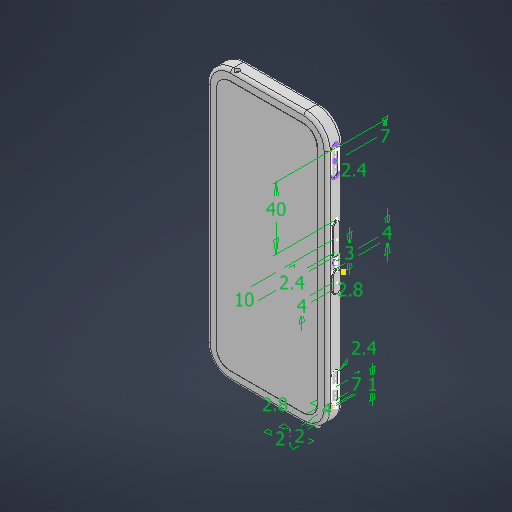
# Autodesk Inventor part: proiect_modelare3D
Saved by Autodesk Inventor 2026.2 (Build 302298000, 298)
## iProperties
Created: 2026-01-05
Part Number: proiect_modelare3D
Material: Generic
Document SubType Name: Modeling
Designer: laura
Density: 1 g/cm^3
Appearance: Default
Author: laura
Autodesk Inventor part; units mm, degrees
ref_plane "YZ Plane" through (0, 0, 0) normal (1, 0, 0) x (0, 1, 0)
ref_plane "XZ Plane" through (0, 0, 0) normal (0, 1, 0) x (-1, 0, 0)
ref_plane "XY Plane" through (0, 0, 0) normal (0, 0, 1) x (1, 0, 0)
sketch "Sketch1" plane through (0, 0, 0) normal (0, 0, 1) x (1, 0, 0)
  line L0 (-23.5, -86.5) -> (23.5, -86.5)
  line L1 (38.5, -71.5) -> (38.5, 71.5)
  line L2 (23.5, 86.5) -> (-23.5, 86.5)
  line L3 (-38.5, 71.5) -> (-38.5, -71.5)
  line L4 (-38.5, -86.5) -> (38.5, 86.5) construction
  line L5 (38.5, -86.5) -> (-38.5, 86.5) construction
  arc A0 (23.5, -86.5) -> (38.5, -71.5) centre (23.5, -71.5) ccw
  arc A1 (-38.5, -71.5) -> (-23.5, -86.5) centre (-23.5, -71.5) ccw
  arc A2 (38.5, 71.5) -> (23.5, 86.5) centre (23.5, 71.5) ccw
  arc A3 (-23.5, 86.5) -> (-38.5, 71.5) centre (-23.5, 71.5) ccw
  point P0 (0, 0)
  dimension "d0" = 173
  dimension "d1" = 77
  dimension "d2" = 15
  dimension "d3" = 15
  dimension "d4" = 15
  constraints: 12 end point, 8 point on circle, 8 point on line, 8 tangent, 4 centre point, 2 midpoint, 2 parallel, 1 equal radius, 1 horizontal, 1 perpendicular
  measures "d0" distance of L5.start L4.end
  measures "d1" distance of L4.end L5.end
  measures "d2" radius of A0
  measures "d3" radius of A1
  measures "d4" radius of A2
extrude "Extrusion1" add sketch "Sketch1" along normal blind 10.3
fillet "Fillet1" radius 2 16 edges at (-34.1066, 82.1066, 0) (-38.5, 0, 0) (-34.1066, -82.1066, 0) (0, -86.5, 0) (34.1066, -82.1066, 0) (38.5, 0, 0) (34.1066, 82.1066, 0) (0, 86.5, 0) (-34.1066, -82.1066, 10.3) (0, -86.5, 10.3) (34.1066, -82.1066, 10.3) (38.5, 0, 10.3) (34.1066, 82.1066, 10.3) (0, 86.5, 10.3) (-34.1066, 82.1066, 10.3) (-38.5, 0, 10.3)
sketch "Sketch2" plane through (0, 0, 10.3) normal (0, 0, 1) x (1, 0, 0)
  line L0 (-23.5, 84.5) -> (23.5, 84.5) projected
  arc A0 (-36.5, -71.5) -> (-23.5, -84.5) centre (-23.5, -71.5) ccw projected
  line L1 (23.5, -84.5) -> (-23.5, -84.5) projected
  arc A1 (23.5, -84.5) -> (36.5, -71.5) centre (23.5, -71.5) ccw projected
  line L2 (36.5, 71.5) -> (36.5, -71.5) projected
  arc A2 (36.5, 71.5) -> (23.5, 84.5) centre (23.5, 71.5) ccw projected
  line L3 (-23.5, 84.5) -> (23.5, 84.5) projected
  arc A3 (-23.5, 84.5) -> (-36.5, 71.5) centre (-23.5, 71.5) ccw projected
  line L4 (-36.5, -71.5) -> (-36.5, 71.5) projected
  arc A4 (32.2574, 71.5) -> (23.5, 80.2574) centre (23.5, 71.5) ccw
  line L5 (32.2574, 71.5) -> (32.2574, -71.5)
  arc A5 (23.5, -80.2574) -> (32.2574, -71.5) centre (23.5, -71.5) ccw
  line L6 (23.5, -80.2574) -> (-23.5, -80.2574)
  arc A6 (-32.2574, -71.5) -> (-23.5, -80.2574) centre (-23.5, -71.5) ccw
  line L7 (-32.2574, -71.5) -> (-32.2574, 71.5)
  arc A7 (-23.5, 80.2574) -> (-32.2574, 71.5) centre (-23.5, 71.5) ccw
  line L8 (-23.5, 80.2574) -> (23.5, 80.2574)
  point P0 (0, 0)
  point P1 (-32.6924, 80.6924)
  point P2 (-29.6924, 77.6924)
  dimension "d8" = 3
  constraints: 10 point on circle, 8 end point, 4 centre point, 7 other
  measures "d8" horizontal distance of point (-32.692, 80.692) point (-29.692, 77.692)
extrude "Extrusion2" add sketch "Sketch2" along normal blind 0.25 contours L5 A5 L6 A6 L7 A7 L8 A4
sketch "Sketch3" plane through (38.5, -71.5, 8.3) normal (1, 0, 0) x (0, 0, -1)
  line L0 (3.15, 100.6) -> (3.15, 85.4) construction
  line L1 (0.75, 100.6) -> (0.75, 85.4)
  line L2 (5.55, 85.4) -> (5.55, 100.6)
  arc A0 (5.55, 100.6) -> (0.75, 100.6) centre (3.15, 100.6) ccw
  arc A1 (0.75, 85.4) -> (5.55, 85.4) centre (3.15, 85.4) ccw
  line L3 (6.3, 143) -> (0, 143) projected
  line L4 (3.15, 142.6032) -> (3.15, 128.6032) construction
  line L5 (5.55, 142.6032) -> (5.55, 128.6032)
  line L6 (0.75, 128.6032) -> (0.75, 142.6032)
  arc A2 (5.55, 142.6032) -> (0.75, 142.6032) centre (3.15, 142.6032) ccw
  arc A3 (0.75, 128.6032) -> (5.55, 128.6032) centre (3.15, 128.6032) ccw
  line L7 (3.15, 17.4) -> (3.15, 3.4) construction
  line L8 (5.55, 17.4) -> (5.55, 3.4)
  line L9 (0.75, 3.4) -> (0.75, 17.4)
  arc A4 (5.55, 17.4) -> (0.75, 17.4) centre (3.15, 17.4) ccw
  arc A5 (0.75, 3.4) -> (5.55, 3.4) centre (3.15, 3.4) ccw
  line L10 (6.3, 0) -> (0, 0) projected
  circle A6 centre (3.15, 80) radius 1.5252
  line L11 (3.15, 73.2) -> (3.15, 65.2) construction
  line L12 (0.35, 73.2) -> (0.35, 65.2)
  line L13 (5.95, 65.2) -> (5.95, 73.2)
  arc A7 (5.95, 73.2) -> (0.35, 73.2) centre (3.15, 73.2) ccw
  arc A8 (0.35, 65.2) -> (5.95, 65.2) centre (3.15, 65.2) ccw
  point P0 (8.3, 71.5)
  point P1 (3.15, 93)
  point P2 (3.15, 83)
  point P3 (3.15, 103)
  point P4 (3.15, 143)
  point P5 (3.15, 143)
  point P6 (3.15, 135.6032)
  point P7 (3.15, 145.0032)
  point P8 (3.15, 143)
  point P9 (3.15, 10.4)
  point P10 (3.15, 1)
  point P11 (3.15, 0)
  point P12 (3.15, 0)
  point P13 (3.15, 69.2)
  point P14 (3.15, 76)
  dimension "d11" = 10
  dimension "d12" = 2.4
  dimension "d13" = 40
  dimension "d14" = 2.4
  dimension "d15" = 2.4
  dimension "d16" = 1
  dimension "d17" = 7
  dimension "d18" = 7
  dimension "d19" = 3
  dimension "d20" = 2.8
  dimension "d21" = 4
  dimension "d22" = 4
  constraints: 32 end point, 21 point on circle, 16 tangent, 9 centre point, 9 midpoint, 5 vertical alignment, 4 parallel, 4 vertical
  measures "d11" distance of point (3.15, 83) point (3.15, 93)
  measures "d12" distance of L0.end point (3.15, 83)
  measures "d13" distance of point (3.15, 103) point (3.15, 143)
  measures "d14" radius of A3
  measures "d15" radius of A4
  measures "d16" distance of point (3.15, 0) point (3.15, 1)
  measures "d17" distance of L7.end point (3.15, 10.4)
  measures "d18" distance of L4.start point (3.15, 135.603)
  measures "d19" distance of point (3.15, 83) A6.centre
  measures "d20" radius of A8
  measures "d21" distance of L11.end point (3.15, 69.2)
  measures "d22" distance of point (3.15, 76) A6.centre
extrude "Extrusion3" cut sketch "Sketch3" against normal blind 1 contours A2 L5 A3 L6 L3 | L3 A2 | L8 A5 L9 A4 | A6
extrude "Extrusion4" add sketch "Sketch3" along normal blind 1 contours A0 L2 A1 L1 | A7 L13 A8 L12
fillet "Fillet2" radius 0.4 27 edges at (38.5, 31.5, 5.15) (38.5, 21.5, 2.75) (38.5, 11.5, 5.15) (38.5, 21.5, 7.55) (38.5, -2.3, 2.35) (38.5, -9.1, 5.15) (38.5, -2.3, 7.95) (38.5, 4.5, 5.15) (38.5, 71.3023, 7.5417) (38.3656, 73.5032, 5.15) (38.5, 71.3023, 2.7583) (38.5, 64.1032, 2.75) (38.5, 54.7032, 5.15) (38.5, 64.1032, 7.55) (38.5, 8.5, 6.6752) (38.5, -51.7, 5.15) (38.5, -61.1, 2.75) (38.5, -70.5, 5.15) (38.5, -61.1, 7.55) (39.5, -9.1, 5.15) (39.5, -2.3, 2.35) (39.5, 4.5, 5.15) (39.5, -2.3, 7.95) (39.5, 31.5, 5.15) (39.5, 21.5, 7.55) (39.5, 11.5, 5.15) (39.5, 21.5, 2.75)
sketch "Sketch4" plane through (-38.5, -71.5, 8.3) normal (-1, 0, 0) x (0, 0, 1)
  line L0 (-5.95, 65.2) -> (-5.95, 73.2) projected
  arc A0 (-5.95, 65.2) -> (-0.35, 65.2) centre (-3.15, 65.2) ccw projected
  arc A1 (-0.35, 73.2) -> (-5.95, 73.2) centre (-3.15, 73.2) ccw projected
  line L1 (-0.35, 73.2) -> (-0.35, 65.2) projected
  line L2 (-5.95, 65.2) -> (-5.95, 73.2) projected
  point P0 (-8.3, 71.5)
extrude "Extrusion5" cut sketch "Sketch4" against normal blind 1
sketch "Sketch5" plane through (-23.5, -86.5, 8.3) normal (0, -1, 0) x (1, 0, 0)
  line L0 (46.2, -3.15) -> (38.2, -3.15) construction
  line L1 (46.2, -0.35) -> (38.2, -0.35)
  line L2 (38.2, -5.95) -> (46.2, -5.95)
  arc A0 (46.2, -5.95) -> (46.2, -0.35) centre (46.2, -3.15) ccw
  arc A1 (38.2, -0.35) -> (38.2, -5.95) centre (38.2, -3.15) ccw
  line L3 (47, -6.3) -> (47, 0) projected
  circle A2 centre (51, -3.15) radius 1.4776
  point P0 (23.5, -8.3)
  point P1 (42.2, -3.15)
  point P2 (49, -3.15)
  point P3 (47, -3.15)
  point P4 (47, -3.15)
  point P5 (47, -5.8333)
  point P6 (47, -0.4667)
  dimension "d30" = 2.8
  dimension "d31" = 4
  dimension "d32" = 2
  dimension "d33" = 2
  constraints: 8 end point, 5 point on circle, 4 tangent, 3 centre point, 3 midpoint, 1 horizontal, 1 horizontal alignment, 1 parallel
  measures "d30" radius of A1
  measures "d31" distance of L0.start point (42.2, -3.15)
  measures "d32" distance of point (49, -3.15) point (47, -3.15)
  measures "d33" distance of A2.centre point (49, -3.15)
extrude "Extrusion6" cut sketch "Sketch5" against normal blind 5 contours A0 L3 L2 A1 L1
extrude "Extrusion7" add sketch "Sketch5" against normal blind 5 contours A0 L3 L2 A1 L1 | A0 L3
extrude "Extrusion8" add sketch "Sketch5" against normal blind 2 contours A2
extrude "Extrusion9" add sketch "Sketch5" along normal blind 2 contours A2
sketch "Sketch6" plane through (27.5, -88.5, 5.15) normal (0, -1, 0) x (1, 0, 0)
  circle A0 centre (-48, 0.0384) radius 2
  line L0 (-51, -3.15) -> (-51, 3.15) projected
  line L1 (-4, 5.15) -> (-51, 5.15) projected
  point P0 (-27.5, -5.15)
  point P1 (-51, 0)
  dimension "d42" = 3
  dimension "d43" = 4
  dimension "d54" = 5.1117
  constraints: 1 centre point, 1 midpoint
  measures "d42" horizontal distance of point (-51, 0) A0.centre
  measures "d43" diameter of A0
  measures "d54" distance from line of L1 A0.centre
extrude "Extrusion10" add sketch "Sketch6" against normal blind 5
sketch "Sketch7" plane through (-23.5, 86.5, 8.3) normal (0, 1, 0) x (1, 0, 0)
  circle A0 centre (2.5326, 0) radius 1.5
  point P0 (23.5, 8.3)
  point P1 (0, 0)
  dimension "d46" = 3
  constraints: 1 centre point, 1 horizontal alignment
  measures "d46" diameter of A0
extrude "Extrusion11" cut sketch "Sketch7" against normal blind 2
sketch "Sketch8" plane through (0, 0, 0) normal (0, 0, -1) x (-1, 0, 0)
  point P0 (0, 0)
extrude "Extrusion12" cut sketch "Sketch5" against normal blind 5 contours A2
extrude "Extrusion13" cut sketch "Sketch5" against normal blind 5 contours A0 L3 L2 A1 L1 | A0 L3
fillet "Fillet3" radius 2 1 edges at (-22.5, -88.5, 5.1884)
extrude "Extrusion14" add sketch "Sketch5" against normal blind 5 contours A2
extrude "Extrusion15" cut sketch "Sketch5" against normal blind 5 contours A2
sketch "Sketch9" plane through (0, 0, 0) normal (0, 0, -1) x (-1, 0, 0)
  line L0 (-25.5494, 79.5) -> (13.2729, 79.5)
  line L1 (15.2729, 77.5) -> (15.2729, 66.1634)
  line L2 (-27.5494, 77.5) -> (-27.5494, 63.9636)
  line L3 (-26.3812, 62.1448) -> (-20.9944, 59.6812)
  line L4 (14.582, 64.6513) -> (9.1952, 59.9879)
  line L5 (7.8862, 59.5) -> (-20.1626, 59.5)
  line L6 (-23.5, 84.5) -> (23.5, 84.5) projected
  arc A0 (-27.5494, 63.9636) -> (-26.3812, 62.1448) centre (-25.5494, 63.9636) ccw
  arc A1 (14.582, 64.6513) -> (15.2729, 66.1634) centre (13.2729, 66.1634) ccw
  arc A2 (7.8862, 59.5) -> (9.1952, 59.9879) centre (7.8862, 61.5) ccw
  arc A3 (-20.9944, 59.6812) -> (-20.1626, 59.5) centre (-20.1626, 61.5) ccw
  arc A4 (-25.5494, 79.5) -> (-27.5494, 77.5) centre (-25.5494, 77.5) ccw
  arc A5 (15.2729, 77.5) -> (13.2729, 79.5) centre (13.2729, 77.5) ccw
  circle A6 centre (-19.5494, 70.7318) radius 3.1961
  circle A7 centre (-12.5494, 70.7318) radius 2.85
  circle A8 centre (-5.5494, 70.7318) radius 2.7
  line L7 (2.7729, 70.7318) -> (-1.2271, 70.7318) construction
  line L8 (2.7729, 69.6319) -> (-1.2271, 69.6319)
  line L9 (-1.2271, 71.8317) -> (2.7729, 71.8317)
  arc A9 (2.7729, 69.6319) -> (2.7729, 71.8317) centre (2.7729, 70.7318) ccw
  arc A10 (-1.2271, 71.8317) -> (-1.2271, 69.6319) centre (-1.2271, 70.7318) ccw
  point P0 (0, 0)
  point P1 (-6.1382, 79.5)
  point P2 (-6.1382, 59.5)
  point P3 (-27.5494, 70.7318)
  point P4 (0.7729, 70.7318)
  dimension "d59" = 5
  dimension "d60" = 20
  dimension "d61" = 2
  dimension "d62" = 8
  dimension "d63" = 7
  dimension "d64" = 5.7
  dimension "d65" = 7
  dimension "d66" = 5.4
  dimension "d67" = 1.0999
  dimension "d68" = 4
  dimension "d69" = 14.5
  constraints: 20 end point, 16 point on circle, 16 tangent, 11 centre point, 5 equal radius, 4 midpoint, 3 horizontal, 1 horizontal alignment, 1 parallel, 1 perpendicular
  measures "d59" distance from line of L6 point (-6.138, 79.5)
  measures "d60" distance of point (-6.138, 59.5) point (-6.138, 79.5)
  measures "d61" radius of A0
  measures "d62" distance of A6.centre point (-27.549, 70.732)
  measures "d63" distance of A6.centre A7.centre
  measures "d64" diameter of A7
  measures "d65" distance of A8.centre A7.centre
  measures "d66" diameter of A8
  measures "d67" radius of A10
  measures "d68" distance of L9.start L9.end
  measures "d69" distance from line of L1 point (0.773, 70.732)
extrude "Extrusion16" add sketch "Sketch9" along normal blind 2
fillet "Fillet4" radius 1.5 24 edges at (20.5883, 59.5458, -2) (6.1382, 59.5, -2) (-8.5847, 59.6259, -2) (-11.8886, 62.3196, -2) (-15.092, 65.3322, -2) (-15.2729, 71.8317, -2) (-14.6872, 78.9142, -2) (6.1382, 79.5, -2) (26.9636, 78.9142, -2) (27.5494, 70.7318, -2) (27.2322, 62.8828, -2) (23.6878, 60.913, -2) (-14.6872, 78.9142, 0) (-15.2729, 71.8317, 0) (-15.092, 65.3322, 0) (-11.8886, 62.3196, 0) (-8.5847, 59.6259, 0) (6.1382, 59.5, 0) (20.5883, 59.5458, 0) (23.6878, 60.913, 0) (27.2322, 62.8828, 0) (27.5494, 70.7318, 0) (26.9636, 78.9142, 0) (6.1382, 79.5, 0)
sketch "Sketch10" plane through (0, 0, 0) normal (0, 0, -1) x (-1, 0, 0)
  line L0 (-23.3379, -60.2139) -> (23.5661, -60.2139) construction
  line L1 (23.5661, -60.2139) -> (23.5661, -74.6077) construction
  line L2 (23.5661, -74.6077) -> (-23.3379, -74.6077) construction
  line L3 (-23.3379, -74.6077) -> (-23.3379, -60.2139) construction
  point P0 (0, 0)
  dimension "d0" = 173
  dimension "d1" = 77
  dimension "d2" = 15
  dimension "d3" = 15
  dimension "d4" = 15
  constraints: 2 other
body "Solid1"
